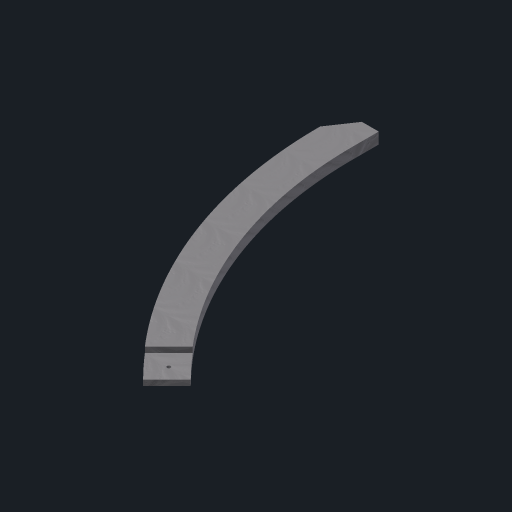
# Autodesk Inventor part: MOLDE_CURVA_1
Saved by Autodesk Inventor 2024.3 (Build 283343000, 343)
## iProperties
Created: 2024-06-12
Part Number: MOLDE_CURVA_1
Material: Steel, Mild, Welded
Document SubType Name: Modeling
Designer: Niler
Density: 7.85 g/cm^3
Appearance: Weld - Steel Mild
Author: Niler
Autodesk Inventor part; units mm, degrees
ref_plane "YZ Plane" through (0, 0, 0) normal (1, 0, 0) x (0, 1, 0)
ref_plane "XZ Plane" through (0, 0, 0) normal (0, 1, 0) x (-1, 0, 0)
ref_plane "XY Plane" through (0, 0, 0) normal (0, 0, 1) x (1, 0, 0)
sketch "Sketch1" plane through (0, 0, 0) normal (0, 1, 0) x (-1, 0, 0)
  arc A0 (350, 0) -> (0, 350) centre (0, 0) ccw
  line L0 (350, 0) -> (350, -22.2048)
  line L1 (0, 350) -> (-24.6, 350)
  line L2 (-24.6, 380) -> (0, 380)
  arc A1 (380, 0) -> (0, 380) centre (0, 0) ccw
  line L3 (380, 0) -> (380, -22.2048)
  line L4 (380, -22.2048) -> (350, -22.2048)
  line L5 (-24.6, 380) -> (-24.6, 350)
  line L6 (380, 0) -> (365, -22.2048)
  line L7 (0, 0) -> (268.7006, 268.7006)
  line L8 (0, 0) -> (0, 91.6225)
  point P0 (247.4874, 247.4874)
  dimension "d0" = 350
  dimension "d1" = 374.6
  dimension "d2" = 30
  constraints: 18 end point, 5 point on circle, 3 vertical, 2 centre point, 2 horizontal, 2 horizontal alignment, 1 coincident, 1 midpoint, 1 tangent, 2 other
  measures "d0" distance from line of L0.start L1
  measures "d1" horizontal distance of L1.end L0.start
  measures "d2" radial gap between concentric circles of A0 A1
extrude "Extrusion1" add sketch "Sketch1" along normal blind 10 contours A0 L7 A1 L6 L4 L0
sketch "Sketch2" plane through (0, 10, 0) normal (0, 1, 0) x (1, 0, 0)
  line L0 (-350, 22.2048) -> (-365, 22.2048) projected
  line L1 (-365, 22.2048) -> (-380, 0) projected
  arc A0 (-380, 0) -> (-268.7006, -268.7006) centre (0, 0) ccw projected
  line L2 (-268.7006, -268.7006) -> (-247.4874, -247.4874) projected
  arc A1 (-350, 0) -> (-247.4874, -247.4874) centre (0, 0) ccw projected
  line L3 (-350, 0) -> (-350, 22.2048) projected
  line L4 (-288.3574, -247.4874) -> (-267.0773, -226.2072)
  constraints: 2 end point, 2 point on circle
extrude "Extrusion2" cut sketch "Sketch2" against normal blind 5 contours A1 L2 A0 L4
sketch "Sketch3" plane through (0, 10, 0) normal (0, 1, 0) x (1, 0, 0)
  arc A0 (-267.0773, -226.2072) -> (-247.4874, -247.4874) centre (0, 0) ccw projected
  line L0 (-288.3574, -247.4874) -> (-267.0773, -226.2072) projected
  arc A1 (-288.3574, -247.4874) -> (-268.7006, -268.7006) centre (0, 0) ccw projected
  line L1 (-247.4874, -247.4874) -> (-268.7006, -268.7006) projected
  circle A2 centre (-267.0773, -247.4874) radius 1.55
  dimension "d7" = 3.1
  constraints: 1 centre point
  measures "d7" diameter of A2
extrude "Extrusion3" cut sketch "Sketch3" against normal through all contours A2
body "Solid1"
